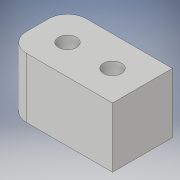
# Autodesk Inventor part: railMount
Saved by Autodesk Inventor 2018 (Build 220112000, 112)
## iProperties
Created: 2020-03-14
Part Number: railMount
Material: Generic
Document SubType Name: Modeling
Designer: natha
Density: 1 g/cm^3
Appearance: Default
Author: natha
Autodesk Inventor part; units mm, degrees
ref_plane "YZ Plane" through (0, 0, 0) normal (1, 0, 0) x (0, 1, 0)
ref_plane "XZ Plane" through (0, 0, 0) normal (0, 1, 0) x (-1, 0, 0)
ref_plane "XY Plane" through (0, 0, 0) normal (0, 0, 1) x (1, 0, 0)
sketch "Sketch1" plane through (0, 0, 0) normal (0, 1, 0) x (-1, 0, 0)
  circle A0 centre (0, 0) radius 6
  line L0 (-20, -20) -> (50, -20)
  line L1 (50, -20) -> (50, 20)
  line L2 (50, 20) -> (-20, 20)
  circle A1 centre (30, 0) radius 6
  line L3 (-20, 20) -> (-20, -20)
  dimension "d0" = 12
  dimension "d1" = 70
  dimension "d2" = 40
  dimension "d3" = 70
  dimension "d4" = 20
  dimension "d7" = 12
  dimension "d8" = 20
  dimension "d9" = 30
  constraints: 8 end point, 2 centre point, 2 perpendicular, 1 coincident, 1 horizontal
  measures "d0" diameter of A0
  measures "d1" distance of L0.start L0.end
  measures "d2" distance of L0.end L1.end
  measures "d3" distance of L1.end L2.end
  measures "d4" distance from line of L0 point (0, 0)
  measures "d7" diameter of A1
  measures "d8" distance from line of L1 A1.centre
  measures "d9" distance of A0.centre A1.centre
extrude "Extrusion1" add sketch "Sketch1" along normal blind 40
fillet "Fillet1" radius 12.7 2 edges at (-50, 20, -20) (-50, 20, 20)
body "Solid1"
